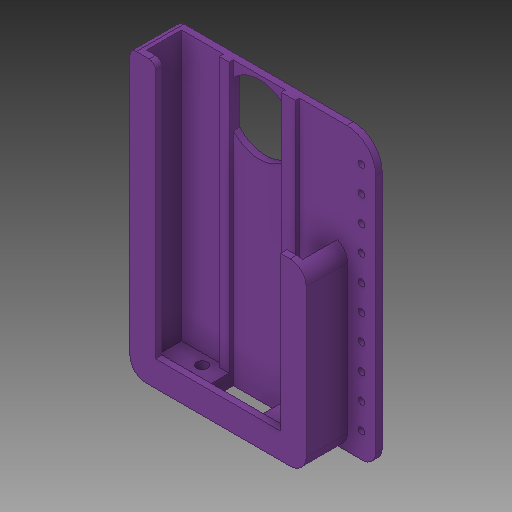
# Autodesk Inventor part: MotoGPhoneHolder
Saved by Autodesk Inventor 2019 (Build 230136000, 136)
## iProperties
Created: 2017-12-05
Part Number: MotoGPhoneHolder
Material: Generic
Document SubType Name: Modeling
Designer: michael.alves
Density: 1 g/cm^3
Appearance: Default
Author: michael.alves
Autodesk Inventor part; units mm, degrees
ref_plane "YZ Plane" through (0, 0, 0) normal (1, 0, 0) x (0, 1, 0)
ref_plane "XZ Plane" through (0, 0, 0) normal (0, 1, 0) x (-1, 0, 0)
ref_plane "XY Plane" through (0, 0, 0) normal (0, 0, 1) x (1, 0, 0)
sketch "Sketch1" plane through (0, 0, 0) normal (0, 0, 1) x (1, 0, 0)
  line L0 (0, 0) -> (87.3125, 0)
  line L1 (87.3125, 0) -> (87.3125, 139.7)
  line L2 (87.3125, 139.7) -> (0, 139.7)
  line L3 (0, 139.7) -> (0, 0)
  dimension "d0" = 87.3125
  dimension "d1" = 139.7
  constraints: 8 end point, 2 parallel, 1 horizontal, 1 perpendicular
  measures "d0" distance of L2.end L1.end
  measures "d1" distance of L1.end L0.end
extrude "body" add sketch "Sketch1" along normal blind 23.622
sketch "Sketch2" plane through (0, 0, 23.622) normal (0, 0, 1) x (1, 0, 0)
  line L0 (87.3125, 139.7) -> (0, 139.7) projected
  line L1 (12.7, 139.7) -> (12.7, 12.7)
  line L2 (12.7, 12.7) -> (74.6125, 12.7)
  line L3 (74.6125, 12.7) -> (74.6125, 139.7)
  line L4 (0, 139.7) -> (0, 0) projected
  line L5 (0, 0) -> (87.3125, 0) projected
  line L6 (87.3125, 0) -> (87.3125, 139.7) projected
  dimension "d4" = 12.7
  dimension "d5" = 12.7
  dimension "d6" = 12.7
  constraints: 6 end point, 2 perpendicular, 2 point on line, 1 vertical
  measures "d4" distance between parallel lines of L4 L1
  measures "d5" distance between parallel lines of L5 L2
  measures "d6" distance between parallel lines of L6 L3
extrude "Extrusion2" cut sketch "Sketch2" against normal blind 16.51 contours L3 L2 L1 L0
sketch "Sketch4" plane through (0, 139.7, 0) normal (0, 1, 0) x (1, 0, 0)
  line L0 (0, 0) -> (0, -23.622) projected
  line L1 (12.7, -23.622) -> (0, -23.622) projected
  line L2 (87.3125, -23.622) -> (74.6125, -23.622) projected
  line L3 (5.08, -3.175) -> (82.2325, -3.175)
  line L4 (82.2325, -3.175) -> (82.2325, -20.447)
  line L5 (82.2325, -20.447) -> (5.08, -20.447)
  line L6 (5.08, -20.447) -> (5.08, -3.175)
  line L7 (87.3125, 0) -> (87.3125, -23.622) projected
  line L8 (12.7, -7.112) -> (74.6125, -7.112) projected
  line L9 (74.6125, -23.622) -> (12.7, -23.622) projected
  line L10 (87.3125, 0) -> (0, 0) projected
  dimension "d9" = 5.08
  dimension "d10" = 5.08
  dimension "d12" = 3.175
  dimension "d15" = 77.1525
  dimension "d17" = 3.175
  constraints: 8 end point, 2 parallel, 1 horizontal, 1 perpendicular
  measures "d9" distance between parallel lines of L7 L4
  measures "d10" distance between parallel lines of L0 L6
  measures "d12" distance between parallel lines of L9 L5
  measures "d15" distance of L3.start L3.end
  measures "d17" distance between parallel lines of L10 L3
extrude "Extrusion3" cut sketch "Sketch4" against normal blind 133.35 contours L3 L4 L5 L6
sketch "Sketch6" plane through (0, 0, 23.622) normal (0, 0, 1) x (1, 0, 0)
  line L0 (5.08, 139.7) -> (5.08, 6.35) projected
  line L1 (12.7, 12.7) -> (12.7, 139.7) projected
  line L2 (12.7, 139.7) -> (0, 139.7) projected
  line L3 (0, 139.7) -> (0, 0) projected
  line L4 (0, 0) -> (87.3125, 0) projected
  line L5 (87.3125, 0) -> (87.3125, 139.7) projected
  line L6 (87.3125, 139.7) -> (74.6125, 139.7) projected
  line L7 (74.6125, 139.7) -> (74.6125, 12.7) projected
  line L8 (74.6125, 12.7) -> (12.7, 12.7) projected
  line L9 (87.3125, 0) -> (87.3125, 139.7) projected
  line L10 (74.6125, 139.7) -> (87.3125, 139.7)
  line L11 (87.3125, 139.7) -> (87.3125, 88.9)
  line L12 (87.3125, 88.9) -> (74.6125, 88.9)
  line L13 (74.6125, 88.9) -> (74.6125, 139.7)
  dimension "d18" = 50.8
  constraints: 8 end point, 2 parallel, 1 horizontal, 1 perpendicular, 1 point on line
  measures "d18" distance of L10.end L11.end
extrude "Extrusion4" cut sketch "Sketch6" against normal up to surface (20.447 mm away) contours L7 L6 L5 L12
sketch "Sketch7" plane through (87.3125, 0, 0) normal (1, 0, 0) x (0, 0, -1)
  line L0 (-3.175, 88.9) -> (-23.622, 88.9) projected
  line L1 (-23.622, 0) -> (-23.622, 88.9) projected
  line L2 (0, 0) -> (-23.622, 0) projected
  line L3 (0, 0) -> (0, 139.7) projected
  line L4 (0, 139.7) -> (-3.175, 139.7) projected
  line L5 (-3.175, 139.7) -> (-3.175, 88.9) projected
  line L6 (0, 0) -> (0, 139.7) projected
  line L7 (-3.175, 139.7) -> (0, 139.7)
  line L8 (0, 139.7) -> (0, 0)
  line L9 (0, 0) -> (-3.175, 0)
  line L10 (-3.175, 0) -> (-3.175, 139.7)
  constraints: 8 end point, 2 parallel, 1 horizontal, 1 perpendicular
extrude "Extrusion5" add sketch "Sketch7" along normal blind 13.97 contours L5 L4 L3 L2 L10
sketch "Sketch8" plane through (0, 139.7, 23.622) normal (0, 1, 0) x (1, 0, 0)
  circle A0 centre (1.2934, 29.8191) radius 10.16
  point P0 (0, 23.622)
  dimension "d23" = 20.32
  constraints: 1 centre point
  measures "d23" diameter of A0
extrude "Extrusion6" add sketch "Sketch8" against normal blind 139.7
sketch "Sketch9" plane through (0, 139.7, 23.622) normal (0, 1, 0) x (1, 0, 0)
  arc A0 (9.3446, 23.622) -> (0, 19.7418) centre (1.2934, 29.8191) ccw projected
  circle A1 centre (1.2934, 29.8191) radius 6.35
  point P0 (0, 23.622)
  dimension "d57" = 12.7
  constraints: 1 centre point, 1 coincident
  measures "d57" diameter of A1
extrude "Extrusion7" cut sketch "Sketch9" against normal blind 88.9
fillet "Fillet1" radius 14.2875 1 edges at (101.2825, 139.7, 1.5875)
fillet "Fillet2" radius 7.9375 1 edges at (0, 0, 13.7511)
fillet "Fillet3" radius 7.9375 2 edges at (87.3125, 0, 13.3985) (87.3125, 88.9, 13.3985)
hole "Hole1" at (94.2975, 12.4085, 3.175) direction (0, 0, -1) diameter 3.302 end through all
pattern_linear "Rectangular Pattern1" count 10 spacing 12.7 along (0, 1, 0) of "Hole1"
sketch "Sketch13" plane through (101.2825, 0, 0) normal (0, -1, 0) x (1, 0, 0)
  line L0 (-26.67, 20.447) -> (-88.5825, 20.447) projected
  line L1 (-96.0661, 3.175) -> (-19.05, 3.175) projected
  line L2 (-70.485, 20.447) -> (-44.7675, 20.447)
  line L3 (-44.7675, 20.447) -> (-44.7675, 3.175)
  line L4 (-44.7675, 3.175) -> (-70.485, 3.175)
  line L5 (-70.485, 3.175) -> (-70.485, 20.447)
  line L6 (-21.9075, 23.622) -> (-21.9075, 3.175) projected
  line L7 (-93.345, 1.4894) -> (-93.345, 23.622) projected
  point P0 (-101.2825, 0)
  point P1 (-96.2025, 3.175)
  point P2 (-93.345, 0)
  dimension "d44" = 22.86
  dimension "d45" = 22.86
  constraints: 8 end point, 2 parallel, 2 point on line, 1 horizontal, 1 perpendicular
  measures "d44" distance between parallel lines of L6 L3
  measures "d45" distance between parallel lines of L7 L5
extrude "Extrusion8" cut sketch "Sketch13" against normal up to next
sketch "Sketch14" plane through (0, 139.7, 3.8802) normal (-1, 0, 0) x (0, 0, 1)
  point P0 (-3.8802, -139.7)
fillet "Fillet4" radius 6.35 1 edges at (101.2825, 0, 1.5875)
fillet "Fillet5" radius 3.175 1 edges at (0, 139.7, 13.7511)
fillet "Fillet6" radius 3.175 1 edges at (12.7, 139.7, 22.0345)
sketch "Sketch18" plane through (5.2164, 6.35, 3.175) normal (0, 0, 1) x (1, 0, 0)
  line L0 (41.021, 167.6656) -> (41.021, -87.2653) construction
  line L1 (82.0961, 1.5875) -> (82.0961, 74.6125) projected
  line L2 (0, 133.35) -> (0, 0) projected
  line L3 (4.1283, 133.35) -> (81.7786, 133.35) projected
  line L4 (20.574, 133.35) -> (61.468, 133.35)
  line L5 (61.468, 133.35) -> (61.468, 0)
  line L6 (61.468, 0) -> (20.574, 0)
  line L7 (20.574, 0) -> (20.574, 133.35)
  point P0 (-5.2164, -6.35)
  point P1 (41.021, 3.169)
  dimension "d63" = 41.0752
  dimension "d64" = 41.021
  dimension "d65" = 20.447
  dimension "d66" = 20.447
  constraints: 10 end point, 2 parallel, 1 horizontal, 1 perpendicular, 1 point on line, 1 vertical
  measures "d63" distance between parallel lines of L0 L1
  measures "d64" distance between parallel lines of L2 L0
  measures "d65" distance between parallel lines of L5 L0
  measures "d66" distance between parallel lines of L0 L7
extrude "Extrusion13" add sketch "Sketch18" along normal blind 2.032
sketch "Sketch19" plane through (30.7975, 6.35, 3.175) normal (0, -1, 0) x (1, 0, 0)
  line L0 (0, 2.032) -> (0, 0) projected
  line L1 (25.7175, 0) -> (0, 0) projected
  line L2 (25.7175, 0) -> (25.7175, 2.032) projected
  line L3 (0, 2.032) -> (25.7175, 2.032) projected
  point P0 (-30.7975, -3.175)
extrude "Extrusion14" cut sketch "Sketch19" against normal up to next
sketch "Sketch20" plane through (5.2164, 6.35, 5.207) normal (0, 0, 1) x (1, 0, 0)
  line L0 (61.468, 133.35) -> (51.2986, 133.35) projected
  line L1 (61.468, 0) -> (51.2986, 0) projected
  line L2 (61.468, 133.35) -> (58.356, 133.35)
  line L3 (58.356, 133.35) -> (58.356, 0)
  line L4 (58.356, 0) -> (61.468, 0)
  line L5 (61.468, 0) -> (61.468, 133.35)
  point P0 (-5.2164, -6.35)
  constraints: 8 end point, 2 parallel, 1 horizontal, 1 perpendicular, 1 point on line
extrude "Extrusion15" cut sketch "Sketch20" against normal up to surface (2.032 mm away)
sketch "Sketch21" plane through (7.9375, 0, 1.4894) normal (0, -1, 0) x (1, 0, 0)
  line L0 (0, 0) -> (0, 22.1326) projected
  line L1 (0, 22.1326) -> (71.4375, 22.1326) projected
  line L2 (86.995, 1.6856) -> (86.995, -1.4894) projected
  line L3 (71.4375, 1.6856) -> (86.995, 1.6856) projected
  line L4 (71.4375, 22.1326) -> (71.4375, 1.6856) projected
  line L5 (0, 22.1326) -> (71.4375, 22.1326) projected
  line L6 (0, 0) -> (0, 22.1326) projected
  arc A0 (0, 0) -> (1.4071, -1.4894) centre (-6.6441, -7.6865) ccw projected
  line L7 (1.4071, -1.4894) -> (86.995, -1.4894) projected
  line L8 (48.5775, 1.6856) -> (22.86, 1.6856) projected
  line L9 (22.86, 1.6856) -> (22.86, 18.9576) projected
  line L10 (22.86, 18.9576) -> (48.5775, 18.9576) projected
  line L11 (48.5775, 18.9576) -> (48.5775, 1.6856) projected
  line L12 (71.4375, 22.1326) -> (71.4375, 1.6856) projected
  line L13 (74.295, 18.9576) -> (48.5775, 18.9576) projected
  circle A1 centre (12.7186, 15.1586) radius 2.7198
  line L14 (-18.0276, 11.0663) -> (85.9797, 11.0663) construction
  line L15 (35.7124, 37.2023) -> (35.7124, -22.0269) construction
  circle A2 centre (12.7186, 6.974) radius 2.7198
  circle A3 centre (58.7062, 15.1586) radius 2.7198
  circle A4 centre (58.7062, 6.974) radius 2.7198
  line L16 (22.86, 18.9576) -> (-2.8575, 18.9576) projected
  line L17 (86.995, 1.6856) -> (86.995, -1.4894) projected
  line L18 (71.4375, 1.6856) -> (86.995, 1.6856) projected
  line L19 (71.4375, 22.1326) -> (71.4375, 1.6856) projected
  line L20 (0, 22.1326) -> (71.4375, 22.1326) projected
  line L21 (0, 0) -> (0, 22.1326) projected
  arc A5 (0, 0) -> (1.4071, -1.4894) centre (-6.6441, -7.6865) ccw projected
  line L22 (1.4071, -1.4894) -> (86.995, -1.4894) projected
  line L23 (48.5775, 1.6856) -> (22.86, 1.6856) projected
  line L24 (22.86, 1.6856) -> (22.86, 18.9576) projected
  line L25 (22.86, 18.9576) -> (48.5775, 18.9576) projected
  line L26 (48.5775, 18.9576) -> (48.5775, 1.6856) projected
  point P0 (-7.9375, -1.4894)
  dimension "d73" = 12.8651
  constraints: 4 centre point, 4 end point, 3 symmetric about line, 1 horizontal, 1 vertical, 3 other
  measures "d73" distance between parallel lines of L11 L15
extrude "Extrusion17" cut sketch "Sketch21" against normal up to next contours A1 | A2 | A3 | A4
sketch "Sketch22" plane through (30.7975, 139.7, 3.175) normal (0, 0, 1) x (1, 0, 0)
  circle A0 centre (12.8524, -19.05) radius 17.145
  line L0 (25.7175, 0) -> (25.7175, -133.35) projected
  line L1 (0, 0) -> (25.7175, 0) projected
  point P0 (-30.7975, -139.7)
  dimension "d76" = 34.29
  dimension "d77" = 12.8651
  dimension "d84" = 19.05
  constraints: 1 centre point
  measures "d76" diameter of A0
  measures "d77" distance from line of L0 A0.centre
  measures "d84" distance from line of L1 A0.centre
extrude "Extrusion18" cut sketch "Sketch22" against normal up to next
sketch "Sketch24" plane through (30.7975, 139.7, 3.175) normal (0, 0, -1) x (-1, 0, 0)
  circle A0 centre (-12.8524, -19.05) radius 17.145 projected
  line L0 (-25.7175, -30.3831) -> (-25.7175, -7.7169) projected
  arc A1 (-25.7175, -7.7169) -> (-25.7175, -30.3831) centre (-12.8524, -19.05) ccw
  point P0 (30.7975, -139.7)
  constraints: 2 point on circle, 1 centre point, 1 concentric
extrude "Extrusion19" add sketch "Sketch24" along normal up to surface (3.175 mm away) contours L0 A0 picked at (-27.1441, -19.05)
sketch "Sketch26" plane through (30.7975, 139.7, 3.175) normal (0, 0, -1) x (-1, 0, 0)
  arc A0 (-25.7175, -30.3831) -> (-25.7175, -7.7169) centre (-12.8524, -19.05) ccw projected
  line L0 (0, -30.3975) -> (0, -7.7025) projected
  arc A1 (0, -30.3975) -> (1.0282, -8.9862) centre (-12.8524, -19.05) ccw
  point P0 (30.7975, -139.7)
  constraints: 3 point on circle, 1 centre point, 1 concentric
extrude "Extrusion20" add sketch "Sketch26" along normal up to surface (3.175 mm away)
sketch "Sketch28" plane through (5.08, 139.7, 20.447) normal (0, 1, 0) x (1, 0, 0)
  arc A0 (4.2646, 20.447) -> (-1.905, 16.6598) centre (-3.7866, 26.6441) ccw projected
  line L0 (4.2646, 20.447) -> (81.915, 20.447) projected
  line L1 (-5.08, 16.5668) -> (-5.08, -3.175) projected
  line L2 (-5.08, -3.175) -> (-5.08, 16.5668) projected
  line L3 (-5.08, 16.5668) -> (4.2646, 16.5668)
  line L4 (4.2646, 16.5668) -> (4.2646, 20.447)
  line L5 (4.2646, 20.447) -> (-5.08, 20.447)
  line L6 (-5.08, 20.447) -> (-5.08, 16.5668)
  point P0 (-5.08, 20.447)
  constraints: 8 end point, 2 parallel, 1 horizontal, 1 perpendicular
extrude "Extrusion21" cut sketch "Sketch28" against normal through all contours L5 L6 A0
fillet "Fillet7" radius 3.175 1 edges at (0, 139.7, 1.95)
fillet "Fillet8" radius 7.9375 1 edges at (0, 0, 1.9401)
body "Solid1"
